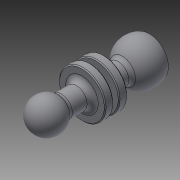
# Autodesk Inventor part: Vertehbrah
Saved by Autodesk Inventor 2014 SP1 (Build 180222100, 222)
## iProperties
Created: 2014-11-05
Part Number: Vertehbrah
Material: Generic
Document SubType Name: Modeling
Designer: rawrdong
Density: 1 g/cm^3
Appearance: Default
Author: rawrdong
Autodesk Inventor part; units mm, degrees
ref_plane "YZ Plane" through (0, 0, 0) normal (1, 0, 0) x (0, 1, 0)
ref_plane "XZ Plane" through (0, 0, 0) normal (0, 1, 0) x (-1, 0, 0)
ref_plane "XY Plane" through (0, 0, 0) normal (0, 0, 1) x (1, 0, 0)
sketch "Sketch1" plane through (0, 0, 0) normal (1, 0, 0) x (0, 1, 0)
  line L0 (-46.83, 0) -> (43.68, 0) projected
  arc A0 (30.75, 9.9593) -> (13.5, 0) centre (25, 0) ccw
  arc A1 (-16.1, 0) -> (-33.9, 0) centre (-25, 0) ccw
  line L1 (-18.2182, 5.7634) -> (-6, 5.7634)
  line L2 (-6, 5.7634) -> (-6, 12.5)
  line L3 (-6, 12.5) -> (-1.5, 12.5)
  line L4 (-1.5, 12.5) -> (-1.5, 7.5)
  line L5 (-1.5, 7.5) -> (1.5, 7.5)
  line L6 (1.5, 7.5) -> (1.5, 12.5)
  line L7 (1.5, 12.5) -> (6, 12.5)
  line L8 (6, 12.5) -> (6, 5.7634)
  line L9 (6, 5.7634) -> (15.0484, 5.7634)
  line L10 (0, 0) -> (0, 20.8147)
  arc A2 (29.55, 7.8808) -> (15.9, 0) centre (25, 0) ccw
  line L11 (-33.9, 0) -> (15.9, 0)
  line L12 (25, 0) -> (30.75, 9.9593)
  dimension "d0" = 50
  dimension "d1" = 3
  dimension "d2" = 7.5
  dimension "d3" = 17.8
  dimension "d4" = 23
  dimension "d5" = 18.2
  dimension "d6" = 12.5
  dimension "d7" = 4.5
  dimension "d8" = 60
  constraints: 24 end point, 8 point on circle, 7 point on line, 6 parallel, 3 centre point, 3 perpendicular, 2 collinear, 1 coincident, 1 symmetric about line, 3 other
  measures "d0" distance of A1.centre A0.centre
  measures "d1" distance between parallel lines of L6 L4
  measures "d2" distance between parallel lines of L0 L5
  measures "d3" diameter of A1
  measures "d4" diameter of A0
  measures "d5" diameter of A2
  measures "d6" distance between parallel lines of L0 L3
  measures "d7" distance between parallel lines of L8 L6
  measures "d8" angle of L11 L12
revolve "Revolution1" add sketch "Sketch1" angle 360 about axis through (0, -10, 0) along (0, 1, 0) contours A1 L0 | A1 L1 L2 L3 L4 L5 L10 L0 | L10 L5 L6 L7 L8 L9 A0 L0 | A0 L12 A2 L0
fillet "Fillet1" radius 3 2 edges at (0, -6, -5.7634) (0, 6, -5.7634)
fillet "Fillet2" radius 3 2 edges at (0, -18.2182, -5.7634) (0, 15.0484, -5.7634)
fillet "Fillet4" radius 0.5 2 edges at (0, 29.55, -7.8808) (0, 30.75, -9.9593)
chamfer "Chamfer1" distance 0.5 angle 45 4 edges at (0, -1.5, -12.5) (0, 1.5, -12.5) (0, 6, -12.5) (0, -6, -12.5)
body "Solid1"
